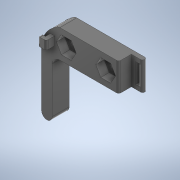
# Autodesk Inventor part: mount_battery
Saved by Autodesk Inventor 2022 (Build 260153000, 153)
## iProperties
Created: 2021-01-30
Part Number: mount_battery
Material: ABS Plastic
Document SubType Name: Modeling
Designer: User
Density: 1.06 g/cm^3
Appearance: Smooth - Black
Author: User
Autodesk Inventor part; units mm, degrees
ref_plane "YZ Plane" through (0, 0, 0) normal (1, 0, 0) x (0, 1, 0)
ref_plane "XZ Plane" through (0, 0, 0) normal (0, 1, 0) x (-1, 0, 0)
ref_plane "Work Plane1" through (0, 0, 0) normal (0, 0, 1) x (1, 0, 0)
sketch "mount_sketch" plane through (0, 0, 0) normal (0, 0, 1) x (1, 0, 0)
  circle A0 centre (42, 55.2584) radius 1.55 projected
  circle A1 centre (28, 55.2584) radius 1.55 projected
  line L0 (45, 60.2584) -> (25, 60.2584)
  line L1 (25, 60.2584) -> (15.4, 52.7584)
  line L2 (15.4, 52.7584) -> (15.4, 29.5584)
  line L3 (15.4, 29.5584) -> (19.4, 29.5584)
  line L4 (19.4, 29.5584) -> (19.4, 48.7584)
  line L5 (19.4, 48.7584) -> (23, 48.7584)
  circle A2 centre (42, -54.7416) radius 1.55 construction
  circle A3 centre (28, -54.7416) radius 1.55 construction
  line L6 (47, -54.627) -> (47, 66.2497) construction
  circle A4 centre (12, 51.2584) radius 1.55 construction
  circle A5 centre (12, -37.8416) radius 1.55 construction
  circle A6 centre (12, -54.7416) radius 1.55 construction
  circle A7 centre (29, -68.7416) radius 1.55 construction
  circle A8 centre (14, -68.7416) radius 1.55 construction
  line L7 (45, 50.2584) -> (25, 50.2584)
  line L8 (25, 50.2584) -> (23, 48.7584)
  line L9 (45, 60.2584) -> (46.5, 60.2584)
  line L10 (46.5, 60.2584) -> (46.5, 50.2584)
  line L11 (46.5, 50.2584) -> (45, 50.2584)
  line L12 (23, 48.7584) -> (23, 58.6959)
  line L13 (35, 55.2584) -> (35, 60.2584)
  line L14 (35, 55.2584) -> (35, 50.2584)
  line L15 (46.5, 60.2584) -> (46.6, 60.2584)
  line L16 (46.6, 60.2584) -> (46.6, 50.2584)
  line L17 (46.6, 50.2584) -> (46.5, 50.2584)
  line L18 (46.6, 60.2584) -> (50.6, 60.2584)
  line L19 (50.6, 60.2584) -> (50.6, 50.2584)
  line L20 (50.6, 50.2584) -> (46.6, 50.2584)
  line L21 (46.6, 50.2584) -> (46.6, 60.2584)
  line L22 (48.1, 58.7584) -> (49.1, 58.7584)
  line L23 (49.1, 58.7584) -> (49.1, 51.7584)
  line L24 (49.1, 51.7584) -> (48.1, 51.7584)
  line L25 (48.1, 51.7584) -> (48.1, 58.7584)
  point P0 (0, 0)
  dimension "d1" = 110
  dimension "d2" = 6.5
  dimension "d3" = 27.6
  dimension "d4" = 4
  dimension "d5" = 14
  dimension "d6" = 5
  dimension "d7" = 19.2
  dimension "d9" = 3.4
  dimension "d13" = 3
  dimension "d30" = 2
  dimension "d32" = 5
  dimension "d62" = 4.5
  dimension "d77" = 4.6
  dimension "d128" = 4
  dimension "d129" = 1.5
  dimension "d130" = 1.5
  dimension "d132" = 7
  dimension "d133" = 1.5
  constraints: 50 end point, 11 perpendicular, 5 horizontal, 4 parallel, 2 midpoint, 2 vertical alignment, 1 point on line, 1 vertical
  measures "d1" distance of A2.centre A0.centre
  measures "d2" distance from line of A0.centre L5
  measures "d3" distance between parallel lines of L6 L4
  measures "d4" distance between parallel lines of L4 L2
  measures "d5" vertical distance of A3.centre A7.centre
  measures "d6" distance from line of L0 A0.centre
  measures "d7" distance between parallel lines of L5 L3
  measures "d9" distance from line of L2 A4.centre
  measures "d13" horizontal distance of L0.end A1.centre
  measures "d30" horizontal distance of L0.end L5.end
  measures "d32" distance from line of L7 A0.centre
  measures "d62" distance from line of L10 A0.centre
  measures "d77" distance from line of L16 A0.centre
  measures "d128" distance of L19.end L20.end
  measures "d129" distance from line of L19 L22.end
  measures "d130" distance from line of L16 L22.start
  measures "d132" distance of L22.end L23.end
  measures "d133" distance between parallel lines of L18 L22
extrude "mount" add sketch "mount_sketch" along normal blind 6
fillet "common" radius 2 2 edges at (25, 60.2584, 3) (25, 50.2584, 3)
sketch "nuts_sketch" plane through (0, 0, 6) normal (0, 0, 1) x (1, 0, 0)
  circle A0 centre (42, 55.2584) radius 1.55 projected
  circle A1 centre (28, 55.2584) radius 1.55 projected
  line L0 (38.4782, 55.2584) -> (40.2391, 58.3084)
  line L1 (40.2391, 58.3084) -> (43.7609, 58.3084)
  line L2 (43.7609, 58.3084) -> (45.5218, 55.2584)
  line L3 (45.5218, 55.2584) -> (43.7609, 52.2084)
  line L4 (43.7609, 52.2084) -> (40.2391, 52.2084)
  line L5 (40.2391, 52.2084) -> (38.4782, 55.2584)
  line L6 (31.5218, 55.2584) -> (29.7609, 52.2084)
  line L7 (29.7609, 52.2084) -> (26.2391, 52.2084)
  line L8 (26.2391, 52.2084) -> (24.4782, 55.2584)
  line L9 (24.4782, 55.2584) -> (26.2391, 58.3084)
  line L10 (26.2391, 58.3084) -> (29.7609, 58.3084)
  line L11 (29.7609, 58.3084) -> (31.5218, 55.2584)
  point P0 (0, 0)
  dimension "d26" = 6.1
  dimension "d27" = 6.1
  constraints: 24 end point, 2 coincident, 2 horizontal alignment, 26 other
  measures "d26" distance between parallel lines of L2 L5
  measures "d27" distance between parallel lines of L8 L11
extrude "nuts" cut sketch "nuts_sketch" against normal blind 3
sketch "Sketch20" plane through (19.4, 29.5584, 0) normal (1, 0, 0) x (0, 0, -1)
  line L0 (-6, 0) -> (-6, 19.2) projected
  line L1 (-6, 0) -> (-6, 19.2)
  line L2 (0, 19.2) -> (-6, 19.2) projected
  line L3 (-6, 19.2) -> (0, 19.2)
  line L4 (0, 0) -> (-6, 0) projected
  line L5 (0, 19.2) -> (0, 0)
  line L6 (0, 0) -> (-6, 0)
  point P0 (0, -29.5584)
  constraints: 8 end point, 2 collinear, 1 perpendicular, 1 vertical
extrude "Extrusion15" add sketch "Sketch20" along normal blind 3.6
sketch "Sketch21" plane through (0, 0, 6) normal (0, 0, 1) x (1, 0, 0)
  line L0 (15.4, 29.5584) -> (23, 29.5584) projected
  line L1 (19.2, 29.5584) -> (19.2, 55.7272)
  line L2 (24.4573, 59.8345) -> (15.4, 52.7584) projected
  line L3 (15.4, 52.7584) -> (15.4, 29.5584) projected
  line L4 (19.2, 29.5584) -> (15.4, 29.5584)
  line L5 (15.4, 29.5584) -> (15.4, 52.7584)
  line L6 (15.4, 52.7584) -> (19.2, 55.7272)
  line L7 (23, 48.7584) -> (24.4667, 49.8584) projected
  line L8 (23, 48.7584) -> (19.2, 48.7584)
  line L9 (23, 48.7584) -> (23, 29.5584) projected
  line L10 (23, 48.7584) -> (23, 58.6959)
  line L11 (19.2, 48.7584) -> (23, 58.6959)
  point P0 (0, 0)
  constraints: 14 end point, 3 point on line, 2 vertical, 1 collinear, 1 horizontal, 1 midpoint, 1 perpendicular
extrude "Extrusion16" cut sketch "Sketch21" against normal blind 6 contours L3 L2 L1 L0
sketch "Sketch22" plane through (0, 0, 6) normal (0, 0, 1) x (1, 0, 0)
  line L0 (23, 48.7584) -> (23, 29.5584) projected
  line L1 (23, 48.7584) -> (23, 58.6959)
  line L2 (24.4573, 59.8345) -> (19.2, 55.7272) projected
  line L3 (23, 48.7584) -> (19.2, 48.7584)
  line L4 (19.2, 29.5584) -> (19.2, 55.7272) projected
  point P0 (0, 0)
  constraints: 4 end point, 2 point on line, 1 perpendicular, 1 vertical
fillet "Fillet12" radius 10 1 edges at (19.2, 55.7272, 3)
fillet "Fillet13" radius 2 1 edges at (23, 48.7584, 3)
fillet "Fillet14" radius 2 2 edges at (23, 29.5584, 3) (19.2, 29.5584, 3)
sketch "Sketch28" plane through (0, 0, 6) normal (0, 0, 1) x (1, 0, 0)
  line L0 (24.4782, 55.2584) -> (26.2391, 58.3084) projected
  line L1 (26.2391, 58.3084) -> (29.7609, 58.3084) projected
  line L2 (29.7609, 58.3084) -> (31.5218, 55.2584) projected
  line L3 (31.5218, 55.2584) -> (29.7609, 52.2084) projected
  line L4 (29.7609, 52.2084) -> (26.2391, 52.2084) projected
  line L5 (26.2391, 52.2084) -> (24.4782, 55.2584) projected
  arc A0 (25.6886, 60.2584) -> (24.4573, 59.8345) centre (25.6886, 58.2584) ccw projected
  line L6 (24.4573, 59.8345) -> (23.0436, 58.73) projected
  arc A1 (23.0436, 58.73) -> (19.2, 50.8497) centre (29.2, 50.8497) ccw projected
  line L7 (19.2, 50.8497) -> (19.2, 31.5484) projected
  arc A2 (19.2, 31.5484) -> (21, 29.5584) centre (21.2, 31.5484) ccw projected
  arc A3 (21, 29.5584) -> (23, 31.5584) centre (21, 31.5584) ccw projected
  line L8 (23, 47.7584) -> (23, 31.5584) projected
  arc A4 (23.8, 49.3584) -> (23, 47.7584) centre (25, 47.7584) ccw projected
  line L9 (23.8, 49.3584) -> (24.4667, 49.8584) projected
  arc A5 (25.6667, 50.2584) -> (24.4667, 49.8584) centre (25.6667, 48.2584) ccw projected
  line L10 (45.5218, 55.2584) -> (43.7609, 52.2084) projected
  line L11 (43.7609, 52.2084) -> (40.2391, 52.2084) projected
  line L12 (40.2391, 52.2084) -> (38.4782, 55.2584) projected
  line L13 (38.4782, 55.2584) -> (40.2391, 58.3084) projected
  line L14 (40.2391, 58.3084) -> (43.7609, 58.3084) projected
  line L15 (43.7609, 58.3084) -> (45.5218, 55.2584) projected
  line L16 (29.7609, 52.2084) -> (26.2391, 52.2084) projected
  line L17 (26.2391, 52.2084) -> (19.2927, 52.2084)
  line L18 (24.4782, 55.2584) -> (22.3512, 55.2584)
  line L19 (22.3512, 55.2584) -> (22.3512, 52.823)
  line L20 (22.3512, 55.2584) -> (20.2243, 55.2584)
  line L21 (22.3512, 55.2584) -> (22.3512, 57.0751)
  line L22 (20.8512, 56.7584) -> (22.3512, 56.7584)
  line L23 (23.8512, 56.7584) -> (23.8512, 53.7584)
  line L24 (23.8512, 53.7584) -> (20.8512, 53.7584)
  line L25 (20.8512, 53.7584) -> (20.8512, 55.2584)
  line L26 (20.8512, 55.2584) -> (20.8512, 56.7584)
  line L27 (22.3512, 56.7584) -> (23.8512, 56.7584)
  line L28 (25.6667, 50.2584) -> (50.6, 50.2584) projected
  line L29 (50.6, 50.2584) -> (50.6, 60.2584) projected
  line L30 (50.6, 60.2584) -> (25.6886, 60.2584) projected
  point P0 (0, 0)
  dimension "d121" = 3
  dimension "d122" = 3
  constraints: 22 end point, 6 parallel, 4 perpendicular, 3 collinear, 2 horizontal, 2 point on circle, 2 point on line, 2 vertical
  measures "d121" distance of L23.start L23.end
  measures "d122" distance of L23.end L24.end
extrude "hook" add sketch "Sketch28" along normal blind 3 contours L23 L24 L19 L18 | L18 L21 L27 L23 | L19 L24 L25 L20 | L20 L26 A1 L22 L21 | L26 L22 A1
sketch "Sketch29" plane through (20.8512, 53.7584, 6) normal (0, -1, 0) x (1, 0, 0)
  line L0 (3, 0) -> (0, 0) projected
  line L1 (3, 0) -> (3, 3) projected
  line L2 (0, 3) -> (3, 3) projected
  line L3 (0, 0) -> (0, 3) projected
  line L4 (0, 0) -> (1.5, 0)
  line L5 (1.5, 0) -> (1.5, 1.7757)
  line L6 (1.5, 1.7757) -> (0, 1.7757)
  line L7 (0, 1.7757) -> (0, 0)
  line L8 (1.5, 1.7757) -> (3, 1.7757)
  line L9 (0, 0) -> (0, 3) projected
  line L10 (0, 1.7757) -> (0, 3)
  point P0 (-20.8512, -6)
  constraints: 12 end point, 2 collinear, 2 parallel, 2 perpendicular, 1 horizontal, 1 point on line
extrude "hook_cutout" cut sketch "Sketch29" against normal through all contours L0 L3 L6 L5
sketch "Sketch33" plane through (0, 0, 6) normal (0, 0, 1) x (1, 0, 0)
  line L0 (49.1, 58.7584) -> (49.1, 51.7584) projected
  line L1 (49.1, 51.7584) -> (48.1, 51.7584) projected
  line L2 (48.1, 51.7584) -> (48.1, 58.7584) projected
  line L3 (48.1, 58.7584) -> (49.1, 58.7584) projected
  line L4 (25.6667, 50.2584) -> (50.6, 50.2584) projected
  line L5 (50.6, 60.2584) -> (25.6886, 60.2584) projected
  line L6 (50.6, 50.2584) -> (46.6, 50.2584)
  line L7 (46.6, 50.2584) -> (46.6, 60.2584)
  line L8 (46.6, 60.2584) -> (50.6, 60.2584)
  line L9 (50.6, 60.2584) -> (50.6, 50.2584)
  point P0 (0, 0)
  dimension "d141" = 4
  constraints: 8 end point, 2 parallel, 1 horizontal, 1 perpendicular, 1 point on line
  measures "d141" distance between parallel lines of L9 L7
extrude "Extrusion25" cut sketch "Sketch33" against normal blind 4.5
fillet "Fillet21" radius 0.75 9 edges at (49.1, 55.2584, 1.5) (50.6, 55.2584, 1.5) (49.1, 55.2584, 0) (50.6, 55.2584, 0) (46.6, 55.2584, 6) (20.8512, 55.2584, 9) (23.8512, 55.2584, 9) (20.8512, 56.7584, 8.3879) (20.8512, 53.7584, 8.3879)
equation "\"d27\" = d26"
equation "\"hook_width\" = 1.5"
equation "\"hook_height\" = 7"
body "Solid1"
